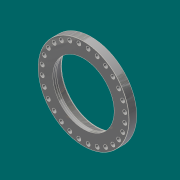
# Autodesk Inventor part: A1-19027-400-06 30in CL300 FF flange
Saved by Autodesk Inventor 2017.3 (Build 213257000, 257)
## iProperties
Created: 2011-05-31
Part Number: A1-19027-400-06 30in CL300 FF flange
Document SubType Name: Modeling
Designer: Graeme_Van_Dongen
Density: 7.85 g/cm^3
Description: 30" CLASS 300 ASME B16.47 Ser.A FFSO FLANGE, A105N, Ø29" BORE
Material: Steel
Mass: 378169 g
Surface Area: 20771.1 cm^2
Volume: 48174.3 cm^3
Appearance: Steel
Author: Graeme_Van_Dongen
Autodesk Inventor part; units mm, degrees
ref_plane "YZ Plane" through (0, 0, 0) normal (1, 0, 0) x (0, 1, 0)
ref_plane "XZ Plane" through (0, 0, 0) normal (0, 1, 0) x (-1, 0, 0)
ref_plane "XY Plane" through (0, 0, 0) normal (0, 0, 1) x (1, 0, 0)
sketch "Sketch1" plane through (0, 0, 0) normal (0, 0, 1) x (1, 0, 0)
  circle A0 centre (0, 0) radius 546.1
  circle A1 centre (0, 0) radius 368.3
  dimension "d0" = 1092.2
  dimension "d1" = 736.6
  constraints: 2 centre point, 2 coincident
  measures "d0" diameter of A0
  measures "d1" diameter of A1
extrude "Extrusion1" add sketch "Sketch1" along normal blind 92.075
sketch "Sketch2" plane through (0, 0, 92.075) normal (0, 0, 1) x (1, 0, 0)
  circle A0 centre (0, 0) radius 368.3 projected
  circle A1 centre (0, 0) radius 546.1 projected
  circle A2 centre (0, 0) radius 428.625
  dimension "d4" = 857.25
  constraints: 1 centre point, 1 coincident
  measures "d4" diameter of A2
extrude "Extrusion2" add sketch "Sketch2" along normal blind 1.5875 contours A2
sketch "Sketch3" plane through (0, 0, 0) normal (0, 0, -1) x (-1, 0, 0)
  circle A0 centre (0, 0) radius 368.3 projected
  circle A1 centre (0, 0) radius 546.1 projected
  circle A2 centre (0, 0) radius 441.325
  dimension "d7" = 882.65
  constraints: 1 centre point, 1 coincident
  measures "d7" diameter of A2
extrude "Extrusion3" add sketch "Sketch3" along normal blind 61.9125 contours A2
sketch "Sketch15" plane through (0, 0, 92.075) normal (0, 0, 1) x (1, 0, 0)
  circle A0 centre (0, 0) radius 428.625 projected
  circle A1 centre (0, 0) radius 546.1 projected
extrude "Extrusion9" add sketch "Sketch15" along normal up to surface (1.5875 mm away)
sketch "Sketch4" plane through (0, 0, 93.6625) normal (0, 0, 1) x (1, 0, 0)
  circle A0 centre (0, 0) radius 428.625 projected
  line L0 (0, -764.54) -> (0, 764.54) projected
  line L1 (-764.54, 0) -> (764.54, 0) projected
  line L2 (0, 0) -> (55.8115, 495.3407) construction
  dimension "d13" = 498.475
  dimension "d14" = 6.429
  constraints: 2 end point
  measures "d13" distance of L2.start L2.end
  measures "d14" angle of L0 L2
hole "Hole1" at (55.8115, 495.3407, 93.6625) direction (0, 0, -1) diameter 47.625 end through all
chamfer "Chamfer3" distance 0.7937 angle 45 2 edges at (55.8115, 519.1532, 0) (55.8115, 519.1532, 93.6625)
pattern_circular "Circular Pattern1" count 28 over 360 about axis through (0, 0, -10) along (0, 0, -1) of "Hole1", "Chamfer3"
chamfer "Chamfer2" distance 1.5875 angle 45 2 edges at (-546.1, 0, 0) (-546.1, 0, 93.6625)
fillet "Fillet2" radius 11.1125 1 edges at (441.325, 0, 0)
chamfer "Chamfer4" distance 1.5875 angle 45 1 edges at (441.325, 0, -61.9125)
sketch "Sketch12" plane through (0, 0, 0) normal (1, 0, 0) x (0, 1, 0)
  line L0 (439.7375, -61.9125) -> (-439.7375, -61.9125) construction
  arc A0 (452.4375, 0) -> (441.325, -11.1125) centre (452.4375, -11.1125) ccw construction
  line L1 (0, -61.9125) -> (0, 93.6625)
  line L2 (368.3, 68.2625) -> (373.0625, 68.2625)
  line L3 (373.0625, 68.2625) -> (373.0625, -61.9125)
  line L4 (373.0625, -61.9125) -> (368.3, -61.9125)
  line L5 (368.3, -61.9125) -> (368.3, 68.2625)
  line L6 (420.6875, -61.9125) -> (420.6875, -55.5625)
  line L7 (420.6875, -55.5625) -> (423.8625, -55.5625)
  line L8 (423.8625, -55.5625) -> (431.8, -49.4718)
  line L9 (431.8, -49.4718) -> (431.8, -39.6875)
  arc A1 (441.325, -27.3908) -> (431.8, -39.6875) centre (444.5, -39.6875) ccw
  line L10 (441.325, -61.9125) -> (420.6875, -61.9125)
  line L11 (368.3, -61.9125) -> (368.3, 93.6625) construction
  line L12 (441.325, -11.1125) -> (441.325, -60.325) construction
  line L13 (441.325, -61.9125) -> (441.325, -27.3908)
  line L14 (373.0625, -61.9125) -> (419.1, -61.9125)
  line L15 (419.1, -61.9125) -> (419.1, -55.5625)
  line L16 (419.1, -55.5625) -> (373.0625, 43.1652)
  dimension "d98" = 863.6
  dimension "d99" = 7.9375
  dimension "d100" = 3.175
  dimension "d101" = 6.35
  dimension "d102" = 37.5
  dimension "d103" = 12.7
  dimension "d104" = 22.225
  dimension "d105" = 9.7843
  dimension "d106" = 746.125
  dimension "d120" = 25.4
  dimension "d134" = 1.5875
  dimension "d135" = 25
  constraints: 28 end point, 8 point on line, 3 parallel, 3 vertical, 2 perpendicular, 2 point on circle, 1 centre point, 1 collinear, 1 horizontal, 1 horizontal alignment, 1 midpoint, 1 tangent
  measures "d98" diameter of L9 L1
  measures "d99" horizontal distance of L7.end L8.end
  measures "d100" distance of L6.end L7.end
  measures "d101" distance of L6.start L6.end
  measures "d102" angle of L7 L8
  measures "d103" radius of A1
  measures "d104" distance from line of L10 A1.centre
  measures "d105" distance of L8.end L9.end
  measures "d106" diameter of L3 L1
  measures "d120" distance from line of L11.end L2
  measures "d134" distance between parallel lines of L6 L15
  measures "d135" angle of L15 L16
revolve "Revolution3" cut sketch "Sketch12" angle 360 about axis through (0, 0, -61.9125) along (0, 0, 1)
fillet "Fillet7" radius 0.7937 1 edges at (0, -373.0625, 68.2625)
chamfer "Chamfer8" distance 0.7937 angle 45 1 edges at (-368.3, 0, 68.2625)
equation "\"d0\" = OD"
equation "\"d1\" = Bore"
equation "\"d2\" = Thickness"
equation "\"d4\" = RFDia"
equation "\"d5\" = RFDepth"
equation "\"d7\" = NeckDia"
equation "\"d8\" = NeckLength"
equation "\"d13\" = 0.5 * BCD"
equation "\"d15\" = HoleDia"
equation "\"d30\" = HoleChamfer"
equation "\"d25\" = RimChamfer"
equation "\"d29\" = NeckFillet"
equation "\"d33\" = NeckChamfer"
equation "\"d98\" = Casing"
equation "\"d106\" = Bore + 2 * Lockstep"
equation "\"OD\" = 1092.2"
equation "\"Bore\" = 736.6"
equation "\"Thickness\" = 92.075"
equation "\"RFDia\" = 857.25"
equation "\"RFDepth\" = 1.5875"
equation "\"HoleDia\" = 47.625"
equation "\"BCD\" = 996.95"
equation "\"NeckDia\" = 882.65"
equation "\"HoleChamfer\" = 0.79375"
equation "\"RimChamfer\" = 1.5875"
equation "\"NeckChamfer\" = 1.5875"
equation "\"NeckFillet\" = 11.1125"
equation "\"Lock\" = 25.4"
equation "\"Lockstep\" = 4.7625"
equation "\"Casing\" = 863.6"
equation "\"Size\" = 762"
equation "\"Wall\" = 9.525"
equation "\"NeckLength\" = 61.9125"
body "Solid1"
